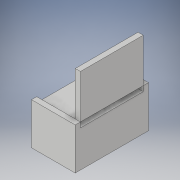
# Autodesk Inventor part: 0 - Fridge
Saved by Autodesk Inventor 2019 (Build 230136000, 136)
## iProperties
Created: 2018-07-18
Part Number: 0 - Fridge
Material: Generic
Document SubType Name: Modeling
Designer: Samuel
Density: 1 g/cm^3
Appearance: Default
Author: Samuel
Autodesk Inventor part; units mm, degrees
ref_plane "YZ Plane" through (0, 0, 0) normal (1, 0, 0) x (0, 1, 0)
ref_plane "XZ Plane" through (0, 0, 0) normal (0, 1, 0) x (-1, 0, 0)
ref_plane "XY Plane" through (0, 0, 0) normal (0, 0, 1) x (1, 0, 0)
sketch "Sketch1" plane through (0, 0, 0) normal (0, 1, 0) x (-1, 0, 0)
  line L0 (0, 0) -> (495, 0)
  line L1 (495, 0) -> (495, -830)
  line L2 (495, -830) -> (0, -830)
  line L3 (0, -830) -> (0, 0)
  dimension "d0" = 495
  dimension "d1" = 830
  constraints: 8 end point, 2 parallel, 1 horizontal, 1 perpendicular
  measures "d0" distance of L1.end L2.end
  measures "d1" distance of L0.end L1.end
extrude "Extrusion1" add sketch "Sketch1" along normal blind 472
sketch "Sketch2" plane through (0, 472, 0) normal (0, 1, 0) x (1, 0, 0)
  line L0 (-495, 0) -> (0, 0) projected
  line L1 (0, 0) -> (0, 830) projected
  line L2 (-495, 0) -> (0, 0)
  line L3 (0, 0) -> (0, 59)
  line L4 (0, 59) -> (-495, 59)
  line L5 (-495, 59) -> (-495, 0)
  line L6 (0, 830) -> (-495, 830) projected
  line L7 (0, 830) -> (-495, 830)
  line L8 (-495, 830) -> (-495, 771)
  line L9 (-495, 771) -> (0, 771)
  line L10 (0, 771) -> (0, 830)
  line L11 (-495, 771) -> (0, 771)
  line L12 (0, 771) -> (0, 59)
  line L13 (0, 59) -> (-495, 59)
  line L14 (-495, 59) -> (-495, 771)
  dimension "d4" = 59
  dimension "d5" = 59
  constraints: 24 end point, 6 parallel, 3 horizontal, 3 perpendicular, 2 point on line
  measures "d4" distance of L3.end L2.end
  measures "d5" distance of L8.end L7.end
extrude "Extrusion2" cut sketch "Sketch2" against normal blind 58.5 contours L14 L9 L1 L4
sketch "Sketch3" plane through (0, 0, 0) normal (1, 0, 0) x (0, 0, -1)
  line L0 (0, 0) -> (0, 472) projected
  line L1 (0, 472) -> (830, 472)
  line L2 (830, 472) -> (830, 967)
  line L3 (830, 967) -> (0, 967)
  line L4 (0, 967) -> (0, 472)
  line L5 (59, 472) -> (59, 413.5) projected
  line L6 (0, 967) -> (59, 967)
  line L7 (59, 967) -> (59, 472)
  line L8 (59, 472) -> (0, 472)
  line L9 (0, 472) -> (0, 967)
  line L10 (771, 472) -> (830, 472)
  line L11 (830, 472) -> (830, 967)
  line L12 (830, 967) -> (771, 967)
  line L13 (771, 967) -> (771, 472)
  line L14 (771, 967) -> (59, 967)
  line L15 (59, 967) -> (59, 472)
  line L16 (59, 472) -> (771, 472)
  line L17 (771, 472) -> (771, 967)
  dimension "d8" = 495
  constraints: 32 end point, 8 parallel, 4 horizontal, 4 perpendicular
  measures "d8" distance of L2.end L1.end
extrude "Extrusion3" add sketch "Sketch3" against normal blind 58.5 contours L7 L3 L13 L1
body "Solid1"
